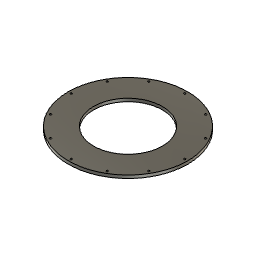
Housing (Autodesk Fusion 360 design; units mm, degrees)
Autodesk Fusion 360 part; units mm, degrees
sketch "Sketch16" plane through (0, 0, 0) normal (0, 0, 1) x (1, 0, 0)
  circle A0 centre (0, 0) radius 100
  circle A1 centre (0, 0) radius 57.5
  circle A2 centre (95, 0) radius 1.5
  dimension "d38" = 115
  dimension "d39" = 200
  dimension "d40" = 3
  dimension "d41" = 95
  constraint coincident A0.centre A1.centre
  measures "d38" diameter of A1
  measures "d39" diameter of A0
  measures "d40" diameter of A2
  measures "d41" distance of A0.centre A2.centre
extrude "Extrude10" add sketch "Sketch16" along normal blind 5
pattern_circular "C-Pattern1" count 12 over 360 about axis through (0, 0, 1.75) along (0, 0, 1) of 1 faces at (96.4981, -0.0748, 3.3333)
sketch "Sketch17" plane through (0, 0, 5) normal (0, 0, 1) x (-1, 0, 0)
  circle A0 centre (-82.2724, 47.5) radius 1.5
  circle A1 centre (-47.5, 82.2724) radius 1.5
  circle A2 centre (0, 95) radius 1.5
  circle A3 centre (47.5, 82.2724) radius 1.5
  circle A4 centre (82.2724, 47.5) radius 1.5
  circle A5 centre (95, 0) radius 1.5
  circle A6 centre (82.2724, -47.5) radius 1.5
  circle A7 centre (47.5, -82.2724) radius 1.5
  circle A8 centre (0, -95) radius 1.5
  circle A9 centre (-47.5, -82.2724) radius 1.5
  circle A10 centre (-82.2724, -47.5) radius 1.5
  circle A11 centre (0, 0) radius 57.5
  circle A12 centre (-95, 0) radius 1.5
  circle A13 centre (0, 0) radius 100
  line L0 (0, 0) -> (47.5, -82.2724) construction
  line L1 (47.5, -82.2724) -> (82.2724, -47.5) construction
  line L2 (82.2724, -47.5) -> (0, 0) construction
  line L3 (64.8862, -64.8862) -> (70.7107, -70.7107) construction
  circle A14 centre (0, 0) radius 90
  circle A15 centre (0, 0) radius 2.1049
  line L4 (70.7107, -70.7107) -> (63.6396, -63.6396)
  line L5 (0, 0) -> (-47.5, -82.2724) construction
  line L6 (-47.5, -82.2724) -> (-82.2724, -47.5) construction
  line L7 (-82.2724, -47.5) -> (0, 0) construction
  line L8 (-64.8862, -64.8862) -> (0, 0) construction
  line L9 (-70.7107, -70.7107) -> (-63.6396, -63.6396)
  line L10 (63.6396, -63.6396) -> (-63.6396, -63.6396) construction
  line L11 (70.7107, -70.7107) -> (-70.7107, -70.7107) construction
  dimension "d46" = 180
  dimension "d66" = 127.2792
  dimension "d67" = 141.4214
  constraint coincident A11.centre A13.centre
  constraint coincident A7.centre L0.end
  constraint coincident A6.centre L1.end
  constraint midpoint L1 L3.start
  constraint coincident A13 L3.end
  constraint perpendicular L1 L3
  constraint coincident A14 L4.end
  constraint perpendicular L1 L4
  constraint coincident A9.centre L5.end
  constraint coincident A10.centre L6.end
  constraint midpoint L6 L8.start
  constraint coincident A13 L9.start
  constraint coincident A14 L9.end
  constraint coincident L8 L9.end
  constraint perpendicular L6 L9
  measures "d46" diameter of A14
  measures "d66" distance of L4.end L9.end
  measures "d67" distance of L3.end L9.start
extrude "Extrude11" [suppressed]
sketch "Sketch18" plane through (0, 0, 5) normal (0, 0, 1) x (-1, 0, 0)
  circle A0 centre (-82.2724, 47.5) radius 1.5
  circle A1 centre (-47.5, 82.2724) radius 1.5
  circle A2 centre (0, 95) radius 1.5
  circle A3 centre (47.5, 82.2724) radius 1.5
  circle A4 centre (82.2724, 47.5) radius 1.5
  circle A5 centre (95, 0) radius 1.5
  circle A6 centre (82.2724, -47.5) radius 1.5
  circle A7 centre (47.5, -82.2724) radius 1.5
  circle A8 centre (0, -95) radius 1.5
  circle A9 centre (-47.5, -82.2724) radius 1.5
  circle A10 centre (-82.2724, -47.5) radius 1.5
  circle A11 centre (0, 0) radius 57.5
  circle A12 centre (-95, 0) radius 1.5
  circle A13 centre (0, 0) radius 100
  line L0 (0, 0) -> (47.5, 82.2724) construction
  line L1 (47.5, 82.2724) -> (82.2724, 47.5) construction
  line L2 (82.2724, 47.5) -> (0, 0) construction
  line L3 (64.8862, 64.8862) -> (0, 0) construction
  line L4 (0, 0) -> (-47.5, 82.2724) construction
  line L5 (-47.5, 82.2724) -> (-82.2724, 47.5) construction
  line L6 (-82.2724, 47.5) -> (0, 0) construction
  line L7 (-64.8862, 64.8862) -> (0, 0) construction
  circle A14 centre (0, 0) radius 90
  circle A15 centre (0, 0) radius 100
  line L8 (70.7107, 70.7107) -> (63.6396, 63.6396)
  line L9 (-70.7107, 70.7107) -> (-63.6396, 63.6396)
  line L10 (-20, 97.9796) -> (20, 97.9796) construction
  line L11 (20, 97.9796) -> (20, 117.9796)
  line L12 (20, 117.9796) -> (-20, 117.9796)
  line L13 (-20, 117.9796) -> (-20, 97.9796)
  line L14 (-20, 97.9796) -> (20, 117.9796) construction
  line L15 (20, 97.9796) -> (-20, 117.9796) construction
  spline S0 degree 5 poles (70.7107, 70.7107) (68.9008, 73.34) (65.2704, 78.4418) (59.7925, 85.6244) (52.4238, 94.254) (43.1033, 103.4152) (33.6745, 110.8808) (24.1439, 116.5701) (14.5261, 120.4049) (4.8489, 122.3332) (-4.8489, 122.3332) (-14.5261, 120.4049) (-24.1439, 116.5701) (-33.6745, 110.8808) (-43.1033, 103.4152) (-52.4238, 94.254) (-59.7925, 85.6244) (-65.2704, 78.4418) (-68.9008, 73.34) (-70.7107, 70.7107) knots 0 0 0 0 0 0 0.066667 0.133333 0.2 0.266667 0.333333 0.4 0.466667 0.533333 0.6 0.666667 0.733333 0.8 0.866667 0.933333 1 1 1 1 1 1
  point P0 (0, 107.9796)
  dimension "d49" = 40
  dimension "d50" = 20
  constraint coincident A11.centre A13.centre
  constraint coincident A3.centre L0.end
  constraint coincident A4.centre L1.end
  constraint midpoint L1 L3.start
  constraint coincident A1.centre L4.end
  constraint coincident A0.centre L5.end
  constraint midpoint L5 L7.start
  constraint coincident A13 L8.start
  constraint coincident L3 L8.end
  constraint coincident A14 L8.end
  constraint perpendicular L1 L8
  constraint coincident A13 L9.start
  constraint coincident A14 L9.end
  constraint coincident L7 L9.end
  constraint perpendicular L5 L9
  constraint horizontal L10
  constraint perpendicular L10 L11
  constraint parallel L10 L12
  constraint parallel L11 L13
  constraint coincident L14 P0
  constraint coincident L15 P0
  constraint coincident A13 L10.start
  constraint coincident A15 L10.end
  measures "d49" distance of L11.end L12.end
  measures "d50" distance of L10 L12
extrude "Extrude12" [suppressed]
sketch "Sketch19" plane through (20, 0, 0) normal (-1, 0, 0) x (0, -1, 0)
  line L0 (97.9796, 5) -> (117.9796, 5)
  line L1 (117.9796, 5) -> (117.9796, 15)
  line L2 (117.9796, 15) -> (97.9796, 15)
  line L3 (97.9796, 15) -> (97.9796, 5)
  line L4 (117.9796, 5) -> (97.9796, 5)
  line L5 (97.9796, 5) -> (97.9796, 15)
  line L6 (97.9796, 15) -> (117.9796, 15)
  line L7 (117.9796, 15) -> (117.9796, 5)
  line L8 (117.9796, 5) -> (70.7107, 5)
  line L9 (70.7107, 5) -> (70.7107, 15)
  line L10 (117.9796, 15) -> (70.7107, 15)
  line L11 (117.9796, 15) -> (117.9796, 5)
  line L12 (70.7107, 5) -> (117.9796, 5)
  line L13 (117.9796, 5) -> (117.9796, 15)
  line L14 (70.7107, 15) -> (117.9796, 15)
  line L15 (70.7107, 15) -> (70.7107, 5)
  line L16 (97.9796, 5) -> (117.9796, 15) construction
  circle A0 centre (107.9796, 10) radius 1.5
  circle A1 centre (107.9796, 10) radius 3
  dimension "d53" = 3
  dimension "d54" = 6
  constraint coincident L0.start L3.end
  constraint coincident L1.end L2.start
  constraint midpoint L16 A0.centre
  constraint concentric A0 A1
  measures "d53" diameter of A0
  measures "d54" diameter of A1
extrude "Extrude13" [suppressed]
extrude "Extrude14" [suppressed]
mirror "Mirror1" [suppressed]
hole "Hole1" [suppressed]
copy_body "Body->Comp1" [suppressed] in component "Component"
